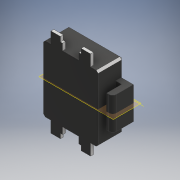
# Autodesk Inventor part: Push-button
Saved by Autodesk Inventor 2017 (Build 210142000, 142)
## iProperties
Created: 2018-07-06
Part Number: Push-button
Material: Generic
Document SubType Name: Modeling
Designer: intelsath
Density: 1 g/cm^3
Appearance: Default
Author: intelsath
Autodesk Inventor part; units mm, degrees
ref_plane "YZ Plane" through (0, 0, 0) normal (1, 0, 0) x (0, 1, 0)
ref_plane "XZ Plane" through (0, 0, 0) normal (0, 1, 0) x (-1, 0, 0)
ref_plane "XY Plane" through (0, 0, 0) normal (0, 0, 1) x (1, 0, 0)
sketch "Sketch1" plane through (0, 0, 0) normal (0, 1, 0) x (-1, 0, 0)
  line L0 (0, 0) -> (-2.9, 0)
  line L1 (-2.9, 0) -> (-2.9, -3.5)
  line L2 (-2.9, -3.5) -> (0, -3.5)
  line L3 (0, -3.5) -> (0, 0)
  dimension "d0" = 2.9
  dimension "d1" = 3.5
  constraints: 8 end point, 2 parallel, 1 horizontal, 1 perpendicular
  measures "d0" distance of L1.end L2.end
  measures "d1" distance of L0.end L1.end
extrude "Extrusion1" add sketch "Sketch1" along normal blind 1.35
sketch "Sketch2" plane through (0, 0, 0) normal (0, -1, 0) x (1, 0, 0)
  line L0 (0.4, -3.5) -> (0.4, -4.1)
  line L1 (0.4, -4.1) -> (0.9, -4.1)
  line L2 (0.9, -4.1) -> (0.9, -3.85)
  line L3 (0.9, -3.85) -> (1.02, -3.85)
  line L4 (1.02, -3.85) -> (1.02, -3.5)
  line L5 (1.02, -3.5) -> (0.4, -3.5)
  line L6 (2.9, -3.5) -> (0, -3.5) projected
  line L7 (0, -3.5) -> (0, 0) construction
  line L8 (0, -1.75) -> (2.9, -1.75) construction
  line L9 (0, 0) -> (2.9, 0) construction
  line L10 (1.45, 0) -> (1.45, -3.5) construction
  line L11 (2.5, -3.5) -> (2.5, -4.1)
  line L12 (2.5, -4.1) -> (2, -4.1)
  line L13 (2, -4.1) -> (2, -3.85)
  line L14 (2, -3.85) -> (1.88, -3.85)
  line L15 (1.88, -3.85) -> (1.88, -3.5)
  line L16 (1.88, -3.5) -> (2.5, -3.5)
  line L17 (2.9, -3.5) -> (2.9, 0) construction
  line L18 (0.4, 0) -> (0.4, 0.6)
  line L19 (0.4, 0.6) -> (0.9, 0.6)
  line L20 (0.9, 0.6) -> (0.9, 0.35)
  line L21 (0.9, 0.35) -> (1.02, 0.35)
  line L22 (1.02, 0.35) -> (1.02, 0)
  line L23 (1.02, 0) -> (0.4, 0)
  line L24 (2.5, 0) -> (2.5, 0.6)
  line L25 (2.5, 0.6) -> (2, 0.6)
  line L26 (2, 0.6) -> (2, 0.35)
  line L27 (2, 0.35) -> (1.88, 0.35)
  line L28 (1.88, 0.35) -> (1.88, 0)
  line L29 (1.88, 0) -> (2.5, 0)
  dimension "d4" = 0.62
  dimension "d5" = 0.5
  dimension "d6" = 0.25
  dimension "d7" = 4.7
  dimension "d8" = 0.86
  constraints: 54 end point, 18 symmetric about line, 3 midpoint, 3 perpendicular, 2 collinear, 2 horizontal, 1 vertical
  measures "d4" distance of L4.end L0.start
  measures "d5" distance of L0.end L1.end
  measures "d6" distance of L1.end L2.end
  measures "d7" distance between parallel lines of L19 L1
  measures "d8" distance between parallel lines of L15 L4
extrude "Extrusion2" add sketch "Sketch2" against normal blind 0.15
chamfer "Chamfer1" distance 0.1 angle 45 8 edges at (2.9, 1.35, -1.75) (1.45, 1.35, 0) (2.9, 0.675, 0) (2.9, 0.675, -3.5) (0, 0.675, 0) (0, 1.35, -1.75) (0, 0.675, -3.5) (1.45, 1.35, -3.5)
ref_plane "Work Plane1" through (0.1, 1.35, -1.75) normal (0, 0, 1) x (1, 0, 0)
sketch "Sketch3" plane through (0.1, 1.35, -1.75) normal (0, 0, 1) x (1, 0, 0)
  line L0 (2.8, -0.125) -> (3.45, -0.125)
  line L1 (3.45, -0.125) -> (3.45, -1.025)
  line L2 (3.25, -1.225) -> (3.125, -1.225)
  line L3 (3.125, -1.225) -> (3.125, -0.425)
  line L4 (3.125, -0.425) -> (2.8, -0.425)
  line L5 (2.8, -0.425) -> (2.8, -0.125)
  line L6 (3.125, -0.125) -> (3.125, -0.425) construction
  arc A0 (3.25, -1.225) -> (3.45, -1.025) centre (3.25, -1.025) ccw
  line L7 (1.48, -0.1666) -> (1.78, -0.1666) construction
  line L8 (2.8, -1.35) -> (2.8, -0.1) projected
  line L9 (2.7, 0) -> (0, 0) projected
  line L10 (2.4, -1.35) -> (2.7, -1.35) projected
  line L11 (-0.1, -0.1) -> (-0.1, -1.35) projected
  dimension "d15" = 0.2
  dimension "d16" = 1.1
  dimension "d17" = 0.3
  dimension "d23" = 0.125
  dimension "d24" = 0.125
  dimension "d25" = 3.55
  constraints: 16 end point, 4 perpendicular, 2 point on circle, 2 tangent, 1 centre point, 1 collinear, 1 horizontal, 1 midpoint, 1 vertical
  measures "d15" radius of A0
  measures "d16" distance between parallel lines of L0 L2
  measures "d17" distance between parallel lines of L0 L4
  measures "d23" distance between parallel lines of L0 L9
  measures "d24" distance between parallel lines of L10 L2
  measures "d25" distance between parallel lines of L11 L1
extrude "Extrusion3" add sketch "Sketch3" along normal mid plane 1.7
equation "\"d23\" = d24"
body "Solid1"
